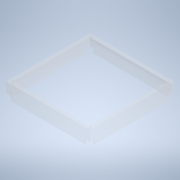
# Autodesk Inventor part: Bottom fabric holder
Saved by Autodesk Inventor 2022 (Build 260153000, 153)
## iProperties
Created: 2021-06-08
Part Number: Bottom fabric holder
Material: PET Plastic
Document SubType Name: Modeling
Designer: benka
Density: 1.541 g/cm^3
Appearance: Polycarbonate - Clear
Author: benka
Autodesk Inventor part; units mm, degrees
ref_plane "YZ Plane" through (0, 0, 0) normal (1, 0, 0) x (0, 1, 0)
ref_plane "XZ Plane" through (0, 0, 0) normal (0, 1, 0) x (-1, 0, 0)
ref_plane "XY Plane" through (0, 0, 0) normal (0, 0, 1) x (1, 0, 0)
sketch "bed" plane through (0, 0, 0) normal (0, 1, 0) x (-1, 0, 0)
  line L0 (59.3441, 94.0804) -> (59.3441, 91.0804)
  line L1 (59.3441, 91.0804) -> (91.3441, 91.0804)
  line L2 (-18.6559, 94.0804) -> (-18.6559, 91.0804)
  line L3 (-18.6559, 91.0804) -> (19.3441, 91.0804)
  line L4 (19.3441, 91.0804) -> (19.3441, 94.0804)
  line L5 (-18.6559, 94.0804) -> (-58.6559, 94.0804)
  line L6 (-58.6559, 94.0804) -> (-58.6559, 91.0804)
  line L7 (59.3441, 94.0804) -> (19.3441, 94.0804)
  line L8 (-58.6559, 91.0804) -> (-90.6559, 91.0804)
  line L9 (59.3441, -93.9196) -> (59.3441, -90.9196)
  line L10 (59.3441, -90.9196) -> (91.3441, -90.9196)
  line L11 (-18.6559, -93.9196) -> (-18.6559, -90.9196)
  line L12 (-18.6559, -90.9196) -> (19.3441, -90.9196)
  line L13 (-58.6559, -93.9196) -> (-58.6559, -90.9196)
  line L14 (59.3441, -93.9196) -> (19.3441, -93.9196)
  line L15 (-18.6559, -93.9196) -> (-58.6559, -93.9196)
  line L16 (-58.6559, -90.9196) -> (-90.6559, -90.9196)
  line L17 (94.3441, 59.0804) -> (91.3441, 59.0804)
  line L18 (94.3441, 59.0804) -> (94.3441, 19.0804)
  line L19 (91.3441, -18.9196) -> (91.3441, 19.0804)
  line L20 (94.3441, -18.9196) -> (91.3441, -18.9196)
  line L21 (94.3441, -58.9196) -> (91.3441, -58.9196)
  line L22 (94.3441, -18.9196) -> (94.3441, -58.9196)
  line L23 (91.3441, 59.0804) -> (91.3441, 91.0804)
  line L24 (91.3441, -58.9196) -> (91.3441, -90.9196)
  line L25 (84.2181, 86.0804) -> (-83.7819, 86.0804)
  line L26 (-85.7819, 84.0804) -> (-85.7819, -83.9196)
  line L27 (-83.7819, -85.9196) -> (84.2181, -85.9196)
  line L28 (86.2181, -83.9196) -> (86.2181, 84.0804)
  arc A0 (86.2181, 84.0804) -> (84.2181, 86.0804) centre (84.2181, 84.0804) ccw
  arc A1 (84.2181, -85.9196) -> (86.2181, -83.9196) centre (84.2181, -83.9196) ccw
  arc A2 (-85.7819, -83.9196) -> (-83.7819, -85.9196) centre (-83.7819, -83.9196) ccw
  arc A3 (-83.7819, 86.0804) -> (-85.7819, 84.0804) centre (-83.7819, 84.0804) ccw
  line L29 (-93.6559, -18.9196) -> (-93.6559, -58.9196)
  line L30 (-93.6559, -58.9196) -> (-90.6559, -58.9196)
  line L31 (-93.6559, -18.9196) -> (-90.6559, -18.9196)
  line L32 (-90.6559, -18.9196) -> (-90.6559, 19.0804)
  line L33 (-90.6559, 19.0804) -> (-93.6559, 19.0804)
  line L34 (-93.6559, 59.0804) -> (-90.6559, 59.0804)
  line L35 (-90.6559, 59.0804) -> (-90.6559, 91.0804)
  line L36 (-93.6559, 59.0804) -> (-93.6559, 19.0804)
  line L37 (-90.6559, -58.9196) -> (-90.6559, -90.9196)
  line L38 (19.3441, -90.9196) -> (19.3441, -93.9196)
  line L39 (91.3441, 19.0804) -> (94.3441, 19.0804)
  circle A4 centre (87.3441, -86.9196) radius 1.5
  circle A5 centre (87.3441, 87.0804) radius 1.5
  circle A6 centre (-86.6559, -86.9196) radius 1.5
  circle A7 centre (-86.6559, 87.0804) radius 1.5
  point P0 (-85.7819, -85.9196)
  point P1 (-85.7819, 86.0804)
  point P2 (86.2181, -85.9196)
  point P3 (-85.1961, 85.4946)
  point P4 (85.6323, 85.4946)
  dimension "d31" = 3
  dimension "d36" = 40
  dimension "d37" = 38
  dimension "d38" = 40
  dimension "d47" = 3
  dimension "d49" = 172
  dimension "d50" = 2
  dimension "d56" = 188
  dimension "d114" = 3
  dimension "d115" = 35
  dimension "d116" = 35
  dimension "d117" = 3
  dimension "d118" = 35
  dimension "d119" = 40
  dimension "d120" = 38
  dimension "d121" = 40
  dimension "d125" = 40
  dimension "d126" = 35
  dimension "d127" = 40
  dimension "d128" = 38
  dimension "d129" = 40
  dimension "d130" = 35
  dimension "d164" = 3
  dimension "d165" = 4
  dimension "d166" = 4
  dimension "d167" = 3
  dimension "d168" = 3
  dimension "d169" = 3
  dimension "d170" = 4
  dimension "d171" = 4
  constraints: 80 end point, 12 collinear, 10 point on circle, 8 centre point, 8 tangent, 6 point on line, 5 horizontal, 3 equal radius, 3 parallel, 2 perpendicular, 4 other
  measures "d31" distance between parallel lines of L3 L5
  measures "d36" distance between parallel lines of L2 L6
  measures "d37" distance between parallel lines of L4 L2
  measures "d38" distance between parallel lines of L0 L4
  measures "d47" distance between parallel lines of L18 L23
  measures "d49" distance of point (-85.782, -85.92) point (-85.782, 86.08)
  measures "d50" radius of A0
  measures "d56" distance between parallel lines of L36 L18
  measures "d114" distance between parallel lines of L35 L36
  measures "d115" distance between parallel lines of L36 L6
  measures "d116" distance between parallel lines of L0 L18
  measures "d117" distance between parallel lines of L8 L5
  measures "d118" distance between parallel lines of L34 L5
  measures "d119" distance between parallel lines of L34 L33
  measures "d120" distance between parallel lines of L31 L33
  measures "d121" distance between parallel lines of L30 L31
  measures "d125" distance between parallel lines of L13 L11
  measures "d126" distance between parallel lines of L17 L7
  measures "d127" distance between parallel lines of L39 L17
  measures "d128" distance between parallel lines of L20 L39
  measures "d129" distance between parallel lines of L21 L20
  measures "d130" distance between parallel lines of L14 L21
  measures "d164" diameter of A4
  measures "d165" distance from line of A4.centre L10
  measures "d166" distance from line of L24 A4.centre
  measures "d167" diameter of A5
  measures "d168" diameter of A6
  measures "d169" diameter of A7
  measures "d170" distance from line of L8 A7.centre
  measures "d171" distance from line of L35 A7.centre
extrude "Extrusion1" add sketch "bed" along normal blind 3
sketch "Sketch10" plane through (93.6559, 0, 59.0804) normal (1, 0, 0) x (0, 0, -1)
  circle A0 centre (59, -13.7365) radius 1.5
  circle A1 centre (-15.1261, -13.7365) radius 1.5
  circle A2 centre (126.8739, -13.7365) radius 1.5
  line L0 (-32, 3) -> (0, 3) projected
  line L1 (0, 0) -> (0, 3) projected
  line L2 (0, 0) -> (40, 0) projected
  line L3 (40, 0) -> (40, 3) projected
  line L4 (40, 3) -> (78, 3) projected
  line L5 (78, 0) -> (78, 3) projected
  line L6 (78, 0) -> (118, 0) projected
  line L7 (118, 0) -> (118, 3) projected
  line L8 (118, 3) -> (150, 3) projected
  line L9 (-35, 3) -> (-32, 3) projected
  line L10 (-35, 3) -> (-35, -7)
  line L11 (-35, -7) -> (-32, -7)
  line L12 (-32, -7) -> (-32, -17)
  line L13 (150, -17) -> (150, -7)
  line L14 (150, -7) -> (153, -7)
  line L15 (150, 3) -> (153, 3) projected
  line L16 (153, -7) -> (153, 3)
  line L17 (-25, -25) -> (-25, -19)
  line L18 (-27, -17) -> (-32, -17)
  line L19 (143, -25) -> (143, -19)
  line L20 (145, -17) -> (150, -17)
  line L21 (-23, -27) -> (141, -27)
  arc A3 (-25, -19) -> (-27, -17) centre (-27, -19) ccw
  arc A4 (-25, -25) -> (-23, -27) centre (-23, -25) ccw
  arc A5 (141, -27) -> (143, -25) centre (141, -25) ccw
  arc A6 (145, -17) -> (143, -19) centre (145, -19) ccw
  point P0 (-25, -27)
  point P1 (-25, -17)
  point P2 (143, -17)
  point P3 (143, -27)
  dimension "d50" = 2
  dimension "d61" = 3
  dimension "d62" = 3
  dimension "d63" = 3
  dimension "d134" = 10
  dimension "d135" = 3
  dimension "d136" = 10
  dimension "d152" = 10
  dimension "d154" = 10
  dimension "d155" = 2
  constraints: 22 end point, 10 point on line, 8 point on circle, 8 tangent, 7 centre point, 3 equal radius, 2 horizontal, 2 perpendicular, 1 vertical
  measures "d61" diameter of A0
  measures "d62" diameter of A1
  measures "d63" diameter of A2
  measures "d134" distance of L9.start L10.end
  measures "d135" distance of L10.end L11.end
  measures "d136" distance of L12.end L11.end
  measures "d152" distance of point (-25, -27) point (-25, -17)
  measures "d154" distance of point (143, -27) point (143, -17)
  measures "d155" radius of A3
extrude "PRINT L" add sketch "Sketch10" against normal blind 3
sketch "Sketch13" plane through (-94.3441, 0, -58.9196) normal (-1, 0, 0) x (0, 0, 1)
  line L0 (-32, -7) -> (-32, -17) projected
  line L1 (-35, -7) -> (-32, -7) projected
  line L2 (-35, 3) -> (-35, -7) projected
  line L3 (150, -7) -> (153, -7) projected
  line L4 (153, -7) -> (153, 3) projected
  circle A0 centre (133.1261, -13.7365) radius 1.5 projected
  circle A1 centre (59, -13.7365) radius 1.5 projected
  circle A2 centre (-8.8739, -13.7365) radius 1.5 projected
  line L5 (-35, 3) -> (-32, 3) projected
  line L6 (-32, 3) -> (0, 3) projected
  line L7 (0, 0) -> (0, 3) projected
  line L8 (0, 0) -> (40, 0) projected
  line L9 (40, 0) -> (40, 3) projected
  line L10 (40, 3) -> (78, 3) projected
  line L11 (78, 0) -> (78, 3) projected
  line L12 (78, 0) -> (118, 0) projected
  line L13 (118, 0) -> (118, 3) projected
  line L14 (118, 3) -> (150, 3) projected
  line L15 (150, 3) -> (153, 3) projected
  line L16 (-32, -17) -> (-27, -17) projected
  arc A3 (-25, -19) -> (-27, -17) centre (-27, -19) ccw projected
  line L17 (-25, -19) -> (-25, -25) projected
  arc A4 (-25, -25) -> (-23, -27) centre (-23, -25) ccw projected
  line L18 (-23, -27) -> (141, -27) projected
  arc A5 (141, -27) -> (143, -25) centre (141, -25) ccw projected
  line L19 (143, -25) -> (143, -19) projected
  arc A6 (145, -17) -> (143, -19) centre (145, -19) ccw projected
  line L20 (145, -17) -> (150, -17) projected
  line L21 (150, -17) -> (150, -7) projected
extrude "Right" add sketch "Sketch13" against normal blind 3
sketch "Sketch14" plane through (-59.3441, 0, 94.0804) normal (0, 0, 1) x (1, 0, 0)
  line L0 (-35, -7) -> (-32, -7) projected
  line L1 (-32, 3) -> (-32, -7) projected
  line L2 (-32, 3) -> (0, 3) projected
  line L3 (0, 0) -> (0, 3) projected
  line L4 (0, 0) -> (40, 0) projected
  line L5 (40, 0) -> (40, 3) projected
  line L6 (40, 3) -> (78, 3) projected
  line L7 (78, 0) -> (78, 3) projected
  line L8 (78, 0) -> (118, 0) projected
  line L9 (118, 3) -> (150, 3) projected
  line L10 (118, 0) -> (118, 3) projected
  line L11 (150, -7) -> (150, 3) projected
  line L12 (153, -7) -> (150, -7) projected
  circle A0 centre (59, -13.7365) radius 1.5
  circle A1 centre (-15.1261, -13.7365) radius 1.5
  circle A2 centre (126.8739, -13.7365) radius 1.5
  line L13 (-35, -17) -> (-35, -7) projected
  line L14 (153, -7) -> (153, -17) projected
  line L15 (-35, -17) -> (-27, -17)
  line L16 (-25, -19) -> (-25, -25)
  line L17 (153, -17) -> (145, -17)
  line L18 (143, -19) -> (143, -25)
  line L19 (-23, -27) -> (141, -27)
  arc A3 (-25, -25) -> (-23, -27) centre (-23, -25) ccw
  arc A4 (-25, -19) -> (-27, -17) centre (-27, -19) ccw
  arc A5 (145, -17) -> (143, -19) centre (145, -19) ccw
  arc A6 (141, -27) -> (143, -25) centre (141, -25) ccw
  point P0 (59.3441, 0)
  point P1 (-25, -27)
  point P2 (-25, -17)
  point P3 (143, -27)
  point P4 (143, -17)
  dimension "d50" = 2
  dimension "d144" = 3
  dimension "d145" = 3
  dimension "d146" = 3
  dimension "d157" = 10
  dimension "d159" = 10
  dimension "d160" = 2
  constraints: 10 end point, 8 point on circle, 8 point on line, 8 tangent, 7 centre point, 3 equal radius, 2 horizontal, 2 perpendicular
  measures "d144" diameter of A0
  measures "d145" diameter of A1
  measures "d146" diameter of A2
  measures "d157" distance of point (-25, -17) point (-25, -27)
  measures "d159" distance of point (143, -27) point (143, -17)
  measures "d160" radius of A3
extrude "PRINT UP" add sketch "Sketch14" against normal blind 3
sketch "Sketch15" plane through (58.6559, 0, -93.9196) normal (0, 0, -1) x (-1, 0, 0)
  circle A0 centre (-8.8739, -13.7365) radius 1.5 projected
  circle A1 centre (59, -13.7365) radius 1.5 projected
  circle A2 centre (133.1261, -13.7365) radius 1.5 projected
  line L0 (-35, -7) -> (-32, -7) projected
  line L1 (-32, 3) -> (-32, -7) projected
  line L2 (-32, 3) -> (0, 3) projected
  line L3 (0, 0) -> (0, 3) projected
  line L4 (0, 0) -> (40, 0) projected
  line L5 (40, 0) -> (40, 3) projected
  line L6 (40, 3) -> (78, 3) projected
  line L7 (78, 0) -> (78, 3) projected
  line L8 (78, 0) -> (118, 0) projected
  line L9 (118, 0) -> (118, 3) projected
  line L10 (118, 3) -> (150, 3) projected
  line L11 (150, 0) -> (150, 3) projected
  line L12 (153, -7) -> (150, -7) projected
  line L13 (150, -7) -> (150, 3) projected
  line L14 (-35, -17) -> (-35, -7) projected
  line L15 (-35, -17) -> (-32, -17) projected
  line L16 (-32, -17) -> (-27, -17) projected
  arc A3 (-25, -19) -> (-27, -17) centre (-27, -19) ccw projected
  line L17 (-25, -19) -> (-25, -25) projected
  arc A4 (-25, -25) -> (-23, -27) centre (-23, -25) ccw projected
  line L18 (-23, -27) -> (141, -27) projected
  arc A5 (141, -27) -> (143, -25) centre (141, -25) ccw projected
  line L19 (143, -25) -> (143, -19) projected
  arc A6 (145, -17) -> (143, -19) centre (145, -19) ccw projected
  line L20 (145, -17) -> (150, -17) projected
  line L21 (153, -17) -> (150, -17) projected
  line L22 (153, -7) -> (153, -17) projected
  point P0 (58.6559, 0)
extrude "Down" add sketch "Sketch15" against normal blind 3
sketch "Sketch16" plane through (-94.3441, 3, 94.0804) normal (0, 1, 0) x (1, 0, 0)
  line L0 (188, 0) -> (0, 0) projected
  line L1 (188, 188) -> (188, 0) projected
  line L2 (188, 188) -> (185, 188) projected
  line L3 (3, 188) -> (185, 188) projected
  line L4 (0, 188) -> (3, 188) projected
  line L5 (0, 0) -> (0, 188) projected
  circle A0 centre (7, 181) radius 1.5 projected
  circle A1 centre (7, 7) radius 1.5 projected
  circle A2 centre (181, 181) radius 1.5 projected
  circle A3 centre (181, 7) radius 1.5 projected
  arc A4 (8.126, 10) -> (10.126, 8) centre (10.126, 10) ccw projected
  line L6 (8.126, 10) -> (8.126, 178) projected
  arc A5 (10.126, 180) -> (8.126, 178) centre (10.126, 178) ccw projected
  line L7 (10.126, 180) -> (178.126, 180) projected
  arc A6 (180.126, 178) -> (178.126, 180) centre (178.126, 178) ccw projected
  line L8 (180.126, 178) -> (180.126, 10) projected
  arc A7 (178.126, 8) -> (180.126, 10) centre (178.126, 10) ccw projected
  line L9 (178.126, 8) -> (10.126, 8) projected
  dimension "d50" = 2
extrude "Extrusion13" add sketch "Sketch16" along normal blind 3
body "Solid1"
